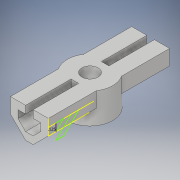
# Autodesk Inventor part: Basic_rail2
Saved by Autodesk Inventor 2018.2 (Build 222227000, 227)
## iProperties
Created: 2018-04-04
Part Number: Basic_rail2
Material: Generic
Document SubType Name: Modeling
Designer: martin
Density: 1 g/cm^3
Appearance: Default
Author: martin
Autodesk Inventor part; units mm, degrees
ref_plane "YZ Plane" through (0, 0, 0) normal (1, 0, 0) x (0, 1, 0)
ref_plane "XZ Plane" through (0, 0, 0) normal (0, 1, 0) x (-1, 0, 0)
ref_plane "XY Plane" through (0, 0, 0) normal (0, 0, 1) x (1, 0, 0)
sketch "Sketch1" plane through (0, 0, 0) normal (0, 0, 1) x (1, 0, 0)
  line L0 (1.5875, 3.175) -> (7.9375, 3.175)
  line L1 (7.9375, 3.175) -> (7.9375, 0)
  line L2 (7.9375, 0) -> (1.5875, 0)
  line L3 (1.5875, 0) -> (1.5875, 3.175)
  line L4 (-7.9375, 3.175) -> (-1.5875, 3.175)
  line L5 (-1.5875, 3.175) -> (-1.5875, 0)
  line L6 (-1.5875, 0) -> (-7.9375, 0)
  line L7 (-7.9375, 0) -> (-7.9375, 3.175)
  line L8 (7.9375, 0) -> (4.7625, 0)
  line L9 (4.7625, 0) -> (4.7625, -3.175)
  line L10 (4.7625, -3.175) -> (7.9375, -3.175)
  line L11 (7.9375, -3.175) -> (7.9375, 0)
  line L12 (-7.9375, 0) -> (-4.7625, 0)
  line L13 (-4.7625, 0) -> (-4.7625, -3.175)
  line L14 (-4.7625, -3.175) -> (-7.9375, -3.175)
  line L15 (-7.9375, -3.175) -> (-7.9375, 0)
  line L16 (-4.7625, -3.175) -> (-1.5875, -6.35)
  line L17 (-1.5875, -6.35) -> (1.5875, -6.35)
  line L18 (1.5875, -6.35) -> (4.7625, -3.175)
  line L19 (7.9375, -3.175) -> (1.5875, -9.525)
  line L20 (1.5875, -9.525) -> (-1.5875, -9.525)
  line L21 (-1.5875, -9.525) -> (-7.9375, -3.175)
  line L22 (-7.9375, -3.175) -> (-4.7625, -3.175)
  point P0 (0, 0)
  dimension "d0" = 6.35
  dimension "d1" = 3.175
  dimension "d2" = 1.5875
  dimension "d3" = 3.175
  dimension "d4" = 6.35
  dimension "d5" = 3.175
  dimension "d6" = 3.175
  dimension "d7" = 4.7625
  dimension "d8" = 4.7625
  dimension "d9" = 3.175
  dimension "d10" = 3.175
  dimension "d11" = 135
  dimension "d12" = 3.175
  constraints: 46 end point, 10 parallel, 6 perpendicular, 5 horizontal, 2 point on line
  measures "d0" distance of L1.end L2.end
  measures "d1" distance of L0.end L1.end
  measures "d2" distance from line of L3 point (0, 0)
  measures "d3" distance from line of L0 point (0, 0)
  measures "d4" distance of L5.end L6.end
  measures "d5" distance of L4.end L5.end
  measures "d6" distance between parallel lines of L5 L3
  measures "d7" distance from line of L13 point (0, 0)
  measures "d8" distance from line of L9 point (0, 0)
  measures "d9" distance from line of L14 point (0, 0)
  measures "d10" horizontal distance of L13.end L16.end
  measures "d11" angle of L14 L16
  measures "d12" distance between parallel lines of L17 L20
extrude "Extrusion1" add sketch "Sketch1" against normal blind 50.8
sketch "Sketch2" plane through (7.9375, -3.175, 0) normal (1, 0, 0) x (0, 0, -1)
  line L0 (0, 3.175) -> (50.8, 3.175) projected
  line L1 (3.175, 3.175) -> (6.35, 3.175)
  line L2 (6.35, 3.175) -> (6.35, -6.35)
  line L3 (6.35, -6.35) -> (3.175, -6.35)
  line L4 (3.175, -6.35) -> (3.175, 3.175)
  line L5 (0, 0) -> (0, 6.35) projected
  line L6 (9.525, 3.175) -> (12.7, 3.175)
  line L7 (12.7, 3.175) -> (12.7, -6.35)
  line L8 (12.7, -6.35) -> (9.525, -6.35)
  line L9 (9.525, -6.35) -> (9.525, 3.175)
  line L10 (15.875, 3.175) -> (19.05, 3.175)
  line L11 (19.05, 3.175) -> (19.05, -6.35)
  line L12 (19.05, -6.35) -> (15.875, -6.35)
  line L13 (15.875, -6.35) -> (15.875, 3.175)
  line L14 (22.225, 3.175) -> (25.4, 3.175)
  line L15 (25.4, 3.175) -> (25.4, -6.35)
  line L16 (25.4, -6.35) -> (22.225, -6.35)
  line L17 (22.225, -6.35) -> (22.225, 3.175)
  line L18 (28.575, 3.175) -> (31.75, 3.175)
  line L19 (31.75, 3.175) -> (31.75, -6.35)
  line L20 (31.75, -6.35) -> (28.575, -6.35)
  line L21 (28.575, -6.35) -> (28.575, 3.175)
  line L22 (34.925, 3.175) -> (38.1, 3.175)
  line L23 (38.1, 3.175) -> (38.1, -6.35)
  line L24 (38.1, -6.35) -> (34.925, -6.35)
  line L25 (34.925, -6.35) -> (34.925, 3.175)
  line L26 (41.275, 3.175) -> (44.45, 3.175)
  line L27 (44.45, 3.175) -> (44.45, -6.35)
  line L28 (44.45, -6.35) -> (41.275, -6.35)
  line L29 (41.275, -6.35) -> (41.275, 3.175)
  line L30 (47.625, 3.175) -> (50.8, 3.175)
  line L31 (50.8, 3.175) -> (50.8, -6.35)
  line L32 (50.8, -6.35) -> (47.625, -6.35)
  line L33 (47.625, -6.35) -> (47.625, 3.175)
  dimension "d15" = 3.175
  dimension "d16" = 3.175
  dimension "d17" = 9.525
  dimension "d18" = 3.175
  dimension "d19" = 3.175
  dimension "d20" = 3.175
  dimension "d21" = 3.175
  dimension "d22" = 3.175
  dimension "d23" = 3.175
  dimension "d24" = 3.175
  dimension "d25" = 3.175
  dimension "d26" = 3.175
  dimension "d27" = 3.175
  dimension "d28" = 3.175
  dimension "d29" = 3.175
  dimension "d30" = 3.175
  dimension "d31" = 3.175
  constraints: 64 end point, 16 parallel, 8 horizontal, 8 perpendicular, 1 point on line
  measures "d15" distance between parallel lines of L5 L4
  measures "d16" distance between parallel lines of L2 L4
  measures "d17" distance between parallel lines of L0 L3
  measures "d18" distance between parallel lines of L7 L9
  measures "d19" distance between parallel lines of L11 L13
  measures "d20" distance between parallel lines of L15 L17
  measures "d21" distance between parallel lines of L19 L21
  measures "d22" distance between parallel lines of L23 L25
  measures "d23" distance between parallel lines of L27 L29
  measures "d24" distance between parallel lines of L9 L2
  measures "d25" distance between parallel lines of L13 L7
  measures "d26" distance between parallel lines of L17 L11
  measures "d27" distance between parallel lines of L21 L15
  measures "d28" distance between parallel lines of L25 L19
  measures "d29" distance between parallel lines of L29 L23
  measures "d30" distance between parallel lines of L31 L33
  measures "d31" distance between parallel lines of L33 L27
extrude "Extrusion2" cut sketch "Sketch2" against normal blind 6.35
sketch "Sketch3" plane through (-7.9375, -3.175, 0) normal (-1, 0, 0) x (0, 0, 1)
  line L0 (-3.175, 3.175) -> (-3.175, 3.175)
  line L1 (-50.8, 3.175) -> (-47.625, 3.175)
  line L2 (-47.625, 3.175) -> (-47.625, -6.35)
  line L3 (-47.625, -6.35) -> (-50.8, -6.35)
  line L4 (-50.8, -6.35) -> (-50.8, 3.175)
  line L5 (-44.45, 3.175) -> (-41.275, 3.175)
  line L6 (-41.275, 3.175) -> (-41.275, -6.35)
  line L7 (-41.275, -6.35) -> (-44.45, -6.35)
  line L8 (-44.45, -6.35) -> (-44.45, 3.175)
  line L9 (-38.1, 3.175) -> (-34.925, 3.175)
  line L10 (-34.925, 3.175) -> (-34.925, -6.35)
  line L11 (-34.925, -6.35) -> (-38.1, -6.35)
  line L12 (-38.1, -6.35) -> (-38.1, 3.175)
  line L13 (-31.75, 3.175) -> (-28.575, 3.175)
  line L14 (-28.575, 3.175) -> (-28.575, -6.35)
  line L15 (-28.575, -6.35) -> (-31.75, -6.35)
  line L16 (-31.75, -6.35) -> (-31.75, 3.175)
  line L17 (-25.4, 3.175) -> (-22.225, 3.175)
  line L18 (-22.225, 3.175) -> (-22.225, -6.35)
  line L19 (-22.225, -6.35) -> (-25.4, -6.35)
  line L20 (-25.4, -6.35) -> (-25.4, 3.175)
  line L21 (-19.05, 3.175) -> (-15.875, 3.175)
  line L22 (-15.875, 3.175) -> (-15.875, -6.35)
  line L23 (-15.875, -6.35) -> (-19.05, -6.35)
  line L24 (-19.05, -6.35) -> (-19.05, 3.175)
  line L25 (-12.7, 3.175) -> (-9.525, 3.175)
  line L26 (-9.525, 3.175) -> (-9.525, -6.35)
  line L27 (-9.525, -6.35) -> (-12.7, -6.35)
  line L28 (-12.7, -6.35) -> (-12.7, 3.175)
  line L29 (-6.35, -6.35) -> (-6.35, 3.175)
  line L30 (-6.35, 3.175) -> (-3.175, 3.175)
  line L31 (-3.175, 3.175) -> (-3.175, -6.35)
  line L32 (-3.175, -6.35) -> (-6.35, -6.35)
  point P0 (0, 3.175)
  point P1 (-3.175, 0)
  dimension "d34" = 3.175
  dimension "d35" = 9.525
  dimension "d36" = 3.175
  dimension "d37" = 3.175
  dimension "d38" = 3.175
  dimension "d39" = 3.175
  dimension "d40" = 3.175
  dimension "d41" = 3.175
  dimension "d42" = 3.175
  dimension "d43" = 3.175
  dimension "d44" = 3.175
  dimension "d45" = 3.175
  dimension "d46" = 3.175
  dimension "d47" = 3.175
  dimension "d48" = 3.175
  dimension "d49" = 3.175
  constraints: 66 end point, 16 parallel, 8 horizontal, 8 perpendicular
  measures "d34" distance between parallel lines of L2 L4
  measures "d35" distance between parallel lines of L0 L3
  measures "d36" distance between parallel lines of L6 L8
  measures "d37" distance between parallel lines of L10 L12
  measures "d38" distance between parallel lines of L14 L16
  measures "d39" distance between parallel lines of L18 L20
  measures "d40" distance between parallel lines of L22 L24
  measures "d41" distance between parallel lines of L26 L28
  measures "d42" distance between parallel lines of L8 L2
  measures "d43" distance between parallel lines of L12 L6
  measures "d44" distance between parallel lines of L16 L10
  measures "d45" distance between parallel lines of L20 L14
  measures "d46" distance between parallel lines of L24 L18
  measures "d47" distance between parallel lines of L28 L22
  measures "d48" distance between parallel lines of L31 L29
  measures "d49" distance between parallel lines of L29 L26
extrude "Extrusion3" cut sketch "Sketch3" against normal blind 6.35
sketch "Sketch4" plane through (-7.9375, 3.175, 0) normal (0, 1, 0) x (1, 0, 0)
  circle A0 centre (7.9375, 25.4) radius 9.525
  point P0 (7.9375, 0)
  dimension "d52" = 19.05
  constraints: 1 centre point
  measures "d52" diameter of A0
extrude "Extrusion4" add sketch "Sketch4" against normal blind 12.7
sketch "Sketch5" plane through (-7.9375, 3.175, 0) normal (0, 1, 0) x (1, 0, 0)
  arc A0 (6.35, 34.7918) -> (6.35, 16.0082) centre (7.9375, 25.4) ccw projected
  circle A1 centre (7.9375, 25.4) radius 3.4036
  point P0 (7.9375, 0)
  dimension "d55" = 6.8072
  constraints: 1 centre point, 1 coincident
  measures "d55" diameter of A1
extrude "Extrusion5" cut sketch "Sketch5" against normal blind 12.7
sketch "Sketch6" plane through (0, 0, 0) normal (0, 0, 1) x (1, 0, 0)
  line L0 (-1.5875, 3.175) -> (-1.5875, 0) projected
  line L1 (-1.5875, 3.175) -> (1.5875, 3.175)
  line L2 (1.5875, 3.175) -> (1.5875, -3.175)
  line L3 (1.5875, -3.175) -> (-1.5875, -3.175)
  line L4 (-1.5875, -3.175) -> (-1.5875, 3.175)
  line L5 (-4.7625, -3.175) -> (-4.7625, 0) projected
  line L6 (-4.7625, 0) -> (4.7625, 0)
  line L7 (4.7625, 0) -> (4.7625, -3.175)
  line L8 (4.7625, -3.175) -> (-4.7625, -3.175)
  line L9 (-4.7625, -3.175) -> (-4.7625, 0)
  point P0 (0, 0)
  constraints: 16 end point, 4 parallel, 2 horizontal, 2 perpendicular
extrude "Extrusion6" cut sketch "Sketch6" against normal blind 19.05
sketch "Sketch7" plane through (0, 0, -50.8) normal (0, 0, -1) x (-1, 0, 0)
  line L0 (-1.5875, 3.175) -> (-1.5875, 0)
  line L1 (-1.5875, 3.175) -> (1.5875, 3.175)
  line L2 (1.5875, 3.175) -> (1.5875, -3.175)
  line L3 (1.5875, -3.175) -> (-1.5875, -3.175)
  line L4 (-1.5875, -3.175) -> (-1.5875, 3.175)
  line L5 (-4.7625, -3.175) -> (-4.7625, 0)
  line L6 (-4.7625, 0) -> (4.7625, 0)
  line L7 (4.7625, 0) -> (4.7625, -3.175)
  line L8 (4.7625, -3.175) -> (-4.7625, -3.175)
  line L9 (-4.7625, -3.175) -> (-4.7625, 0)
  point P0 (0, 0)
  point P1 (0, 0)
  constraints: 20 end point, 4 parallel, 2 horizontal, 2 perpendicular
extrude "Extrusion7" cut sketch "Sketch7" against normal blind 19.05
sketch "Sketch9" plane through (0, 0, 0) normal (0, 0, 1) x (1, 0, 0)
  line L0 (4.7625, 0) -> (1.5875, 0) projected
  line L1 (4.7625, -3.175) -> (4.7625, 0) projected
  line L2 (4.7625, 0) -> (4.7625, -3.175)
  line L3 (1.5875, -6.35) -> (4.7625, -3.175) projected
  line L4 (4.7625, -3.175) -> (1.5875, -6.35)
  line L5 (-1.5875, -6.35) -> (1.5875, -6.35) projected
  line L6 (1.5875, -6.35) -> (-1.5875, -6.35)
  line L7 (-1.5875, -6.35) -> (-4.7625, -3.175) projected
  line L8 (-1.5875, -6.35) -> (-4.7625, -3.175)
  line L9 (-4.7625, -3.175) -> (-4.7625, 0)
  line L10 (-7.9375, 0) -> (-4.7625, 0) projected
  line L11 (-4.7625, 0) -> (-7.9375, 0)
  line L12 (-7.9375, 0) -> (-7.9375, -3.175)
  line L13 (-7.9375, -3.175) -> (-1.5875, -9.525)
  line L14 (-7.0995, -4.013) -> (-7.9375, -3.175) projected
  line L15 (-1.5875, -9.525) -> (1.5875, -9.525) projected
  line L16 (-1.5875, -9.525) -> (1.5875, -9.525)
  line L17 (7.9375, -3.175) -> (1.5875, -9.525) projected
  line L18 (1.5875, -9.525) -> (7.9375, -3.175)
  line L19 (7.9375, 0) -> (7.9375, -3.175) projected
  line L20 (7.9375, -3.175) -> (7.9375, 0)
  line L21 (7.9375, 0) -> (4.7625, 0)
  point P0 (0, 0)
  constraints: 24 end point, 7 collinear, 2 point on line, 1 perpendicular
extrude "Extrusion8" add sketch "Sketch9" against normal blind 50.8
sketch "Sketch12" plane through (7.9375, -3.175, 0) normal (1, 0, 0) x (0, 0, -1)
  line L0 (3.175, 3.175) -> (6.35, 3.175)
  line L1 (0, 3.175) -> (19.05, 3.175) projected
  line L2 (0, 0) -> (17.1511, 0) projected
  line L3 (6.35, 3.175) -> (3.175, 0)
  line L4 (3.175, 0) -> (3.175, 3.175)
  line L5 (0, 0) -> (0, 6.35) projected
  line L6 (9.525, 3.175) -> (3.175, -3.175)
  line L7 (3.175, -3.175) -> (6.35, -3.175)
  line L8 (6.35, -3.175) -> (12.7, 3.175)
  line L9 (0, 3.175) -> (19.05, 3.175) projected
  dimension "d67" = 3.175
  constraints: 12 end point, 1 parallel, 1 perpendicular, 1 point on line
  measures "d67" distance between parallel lines of L5 L4
body "Solid1"
